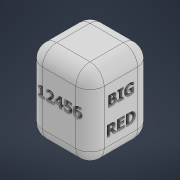
# Autodesk Inventor part: Big Red Basic Capstone
Saved by Autodesk Inventor 2022 (Build 260153000, 153)
## iProperties
Created: 2022-01-25
Part Number: Big Red Basic Capstone
Material: Generic
Document SubType Name: Modeling
Designer: izack
Density: 1 g/cm^3
Appearance: Default
Author: izack
Autodesk Inventor part; units mm, degrees
ref_plane "YZ Plane" through (0, 0, 0) normal (1, 0, 0) x (0, 1, 0)
ref_plane "XZ Plane" through (0, 0, 0) normal (0, 1, 0) x (-1, 0, 0)
ref_plane "XY Plane" through (0, 0, 0) normal (0, 0, 1) x (1, 0, 0)
sketch "Sketch1" plane through (0, 0, 0) normal (0, 1, 0) x (-1, 0, 0)
  line L0 (0, 0) -> (76.2, 0)
  line L1 (76.2, 0) -> (76.2, -76.2)
  line L2 (76.2, -76.2) -> (0, -76.2)
  line L3 (0, -76.2) -> (0, 0)
  dimension "d0" = 76.2
  dimension "d1" = 76.2
  constraints: 8 end point, 2 parallel, 1 horizontal, 1 perpendicular
  measures "d0" distance of L1.end L2.end
  measures "d1" distance of L0.end L1.end
extrude "Extrusion1" add sketch "Sketch1" along normal blind 101.6
shell "Shell1" thickness 12.7 removed faces 1 at (-25.4, 0, -25.4)
fillet "Fillet1" radius 17.4625 20 edges at (-38.1, 88.9, -63.5) (-63.5, 88.9, -38.1) (-63.5, 44.45, -63.5) (-63.5, 44.45, -12.7) (-12.7, 88.9, -38.1) (-38.1, 88.9, -12.7) (-12.7, 44.45, -63.5) (-12.7, 44.45, -12.7) (-38.1, 0, -76.2) (-76.2, 0, -38.1) (-38.1, 0, 0) (0, 0, -38.1) (-76.2, 50.8, -76.2) (-38.1, 101.6, -76.2) (-76.2, 101.6, -38.1) (0, 50.8, -76.2) (-76.2, 50.8, 0) (0, 50.8, 0) (-38.1, 101.6, 0) (0, 101.6, -38.1)
sketch "Sketch2" plane through (-76.2, 17.4625, -17.4625) normal (-1, 0, 0) x (0, 0, 1)
  line L0 (-41.275, 66.675) -> (-41.275, 0) projected
  line L1 (-41.275, 41.2843) -> (0, 41.2843)
  line L2 (0, 41.2843) -> (0, 10.1549)
  line L3 (0, 0) -> (0, 66.675) projected
  line L4 (-41.275, 10.1549) -> (0, 10.1549)
  spline S0 degree 2 poles (-25.8863, 45.1746) (-25.8863, 44.2278) (-26.6067, 42.7972) (-27.2036, 42.3238) knots 0 0 0 1 2 2 2
  spline S1 degree 2 poles (-27.2036, 42.3238) (-27.924, 41.7577) (-29.6325, 41.2843) (-30.9601, 41.2843) knots 0 0 0 1 2 2 2
  line L5 (-30.9601, 41.2843) -> (-36.0339, 41.2843)
  line L6 (-36.0339, 41.2843) -> (-36.0339, 53.9843)
  line L7 (-36.0339, 53.9843) -> (-31.557, 53.9843)
  spline S2 degree 2 poles (-31.557, 53.9843) (-30.1574, 53.9843) (-28.7165, 53.7682) (-28.0887, 53.4286) knots 0 0 0 1 2 2 2
  spline S3 degree 2 poles (-28.0887, 53.4286) (-27.3992, 53.0684) (-26.7302, 51.8333) (-26.7302, 51.0306) knots 0 0 0 1 2 2 2
  spline S4 degree 2 poles (-26.7302, 51.0306) (-26.7302, 50.1043) (-27.6565, 48.6532) (-28.4798, 48.3136) knots 0 0 0 1 2 2 2
  line L8 (-28.4798, 48.3136) -> (-28.4798, 48.2518)
  spline S5 degree 2 poles (-28.4798, 48.2518) (-27.2963, 48.0048) (-25.8863, 46.4713) (-25.8863, 45.1746) knots 0 0 0 1 2 2 2
  spline S6 degree 2 poles (-29.1796, 45.226) (-29.1796, 45.823) (-29.6531, 46.4919) (-30.1265, 46.6669) knots 0 0 0 1 2 2 2
  spline S7 degree 2 poles (-30.1265, 46.6669) (-30.4146, 46.7801) (-31.4335, 46.8007) (-32.2775, 46.8007) knots 0 0 0 1 2 2 2
  line L9 (-32.2775, 46.8007) -> (-32.8641, 46.8007)
  line L10 (-32.8641, 46.8007) -> (-32.8641, 43.6)
  line L11 (-32.8641, 43.6) -> (-32.6891, 43.6)
  spline S8 degree 2 poles (-32.6891, 43.6) (-31.4541, 43.6) (-30.5073, 43.6308) (-30.0133, 43.847) knots 0 0 0 1 2 2 2
  spline S9 degree 2 poles (-30.0133, 43.847) (-29.581, 44.0425) (-29.1796, 44.7629) (-29.1796, 45.226) knots 0 0 0 1 2 2 2
  spline S10 degree 2 poles (-29.9721, 50.4028) (-29.9721, 50.7115) (-30.2911, 51.3599) (-30.6205, 51.504) knots 0 0 0 1 2 2 2
  spline S11 degree 2 poles (-30.6205, 51.504) (-30.9292, 51.6481) (-31.7937, 51.6687) (-32.648, 51.6687) knots 0 0 0 1 2 2 2
  line L12 (-32.648, 51.6687) -> (-32.8641, 51.6687)
  line L13 (-32.8641, 51.6687) -> (-32.8641, 48.9722)
  line L14 (-32.8641, 48.9722) -> (-32.4627, 48.9722)
  spline S12 degree 2 poles (-32.4627, 48.9722) (-31.6497, 48.9722) (-30.991, 49.0031) (-30.6411, 49.1678) knots 0 0 0 1 2 2 2
  spline S13 degree 2 poles (-30.6411, 49.1678) (-30.2603, 49.353) (-29.9721, 49.9808) (-29.9721, 50.4028) knots 0 0 0 1 2 2 2
  line L15 (-17.7352, 41.2843) -> (-24.5689, 41.2843)
  line L16 (-24.5689, 41.2843) -> (-24.5689, 43.497)
  line L17 (-24.5689, 43.497) -> (-22.7473, 43.497)
  line L18 (-22.7473, 43.497) -> (-22.7473, 51.7716)
  line L19 (-22.7473, 51.7716) -> (-24.5689, 51.7716)
  line L20 (-24.5689, 51.7716) -> (-24.5689, 53.9843)
  line L21 (-24.5689, 53.9843) -> (-17.7352, 53.9843)
  line L22 (-17.7352, 53.9843) -> (-17.7352, 51.7716)
  line L23 (-17.7352, 51.7716) -> (-19.5569, 51.7716)
  line L24 (-19.5569, 51.7716) -> (-19.5569, 43.497)
  line L25 (-19.5569, 43.497) -> (-17.7352, 43.497)
  line L26 (-17.7352, 43.497) -> (-17.7352, 41.2843)
  spline S14 degree 2 poles (-5.0146, 42.0047) (-5.8483, 41.6651) (-8.5138, 41.0167) (-9.8106, 41.0167) knots 0 0 0 1 2 2 2
  spline S15 degree 2 poles (-9.8106, 41.0167) (-12.8055, 41.0167) (-16.3561, 44.4748) (-16.3561, 47.6446) knots 0 0 0 1 2 2 2
  spline S16 degree 2 poles (-16.3561, 47.6446) (-16.3561, 50.6292) (-12.8055, 54.2313) (-9.718, 54.2313) knots 0 0 0 1 2 2 2
  spline S17 degree 2 poles (-9.718, 54.2313) (-8.1228, 54.2313) (-6.1262, 53.6241) (-5.0661, 53.1095) knots 0 0 0 1 2 2 2
  line L27 (-5.0661, 53.1095) -> (-5.0661, 50.1249)
  line L28 (-5.0661, 50.1249) -> (-5.3543, 50.1249)
  spline S18 degree 2 poles (-5.3543, 50.1249) (-5.5807, 50.2999) (-6.4452, 50.9688) (-6.8569, 51.1953) knots 0 0 0 1 2 2 2
  spline S19 degree 2 poles (-6.8569, 51.1953) (-7.3303, 51.4731) (-8.5859, 51.8642) (-9.2857, 51.8642) knots 0 0 0 1 2 2 2
  spline S20 degree 2 poles (-9.2857, 51.8642) (-10.0988, 51.8642) (-11.447, 51.3496) (-11.9719, 50.8248) knots 0 0 0 1 2 2 2
  spline S21 degree 2 poles (-11.9719, 50.8248) (-12.4762, 50.3102) (-13.0628, 48.7355) (-13.0628, 47.6961) knots 0 0 0 1 2 2 2
  spline S22 degree 2 poles (-13.0628, 47.6961) (-13.0628, 45.4731) (-10.8295, 43.353) (-8.9049, 43.353) knots 0 0 0 1 2 2 2
  spline S23 degree 2 poles (-8.9049, 43.353) (-8.73, 43.353) (-8.2771, 43.3735) (-8.1022, 43.3838) knots 0 0 0 1 2 2 2
  line L29 (-8.1022, 43.3838) -> (-8.1022, 45.8847)
  line L30 (-8.1022, 45.8847) -> (-10.5619, 45.8847)
  line L31 (-10.5619, 45.8847) -> (-10.5619, 48.2621)
  line L32 (-10.5619, 48.2621) -> (-5.0146, 48.2621)
  line L33 (-5.0146, 48.2621) -> (-5.0146, 42.0047)
  line L34 (-25.912, 10.1549) -> (-29.792, 10.1549)
  line L35 (-29.792, 10.1549) -> (-33.3221, 14.817)
  line L36 (-33.3221, 14.817) -> (-34.4747, 14.817)
  line L37 (-34.4747, 14.817) -> (-34.4747, 10.1549)
  line L38 (-34.4747, 10.1549) -> (-37.6446, 10.1549)
  line L39 (-37.6446, 10.1549) -> (-37.6446, 22.8549)
  line L40 (-37.6446, 22.8549) -> (-32.5399, 22.8549)
  spline S24 degree 2 poles (-32.5399, 22.8549) (-31.4798, 22.8549) (-29.9155, 22.5873) (-29.2465, 22.1756) knots 0 0 0 1 2 2 2
  spline S25 degree 2 poles (-29.2465, 22.1756) (-28.5673, 21.7434) (-27.7645, 20.3952) (-27.7645, 19.366) knots 0 0 0 1 2 2 2
  spline S26 degree 2 poles (-27.7645, 19.366) (-27.7645, 17.9149) (-29.0819, 16.0932) (-30.1831, 15.558) knots 0 0 0 1 2 2 2
  line L41 (-30.1831, 15.558) -> (-25.912, 10.1549)
  spline S27 degree 2 poles (-31.0373, 18.9646) (-31.0373, 19.4483) (-31.4078, 20.1379) (-31.8298, 20.3231) knots 0 0 0 1 2 2 2
  spline S28 degree 2 poles (-31.8298, 20.3231) (-32.1282, 20.4466) (-32.8589, 20.5187) (-33.4044, 20.5187) knots 0 0 0 1 2 2 2
  line L42 (-33.4044, 20.5187) -> (-34.4747, 20.5187)
  line L43 (-34.4747, 20.5187) -> (-34.4747, 17.1018)
  line L44 (-34.4747, 17.1018) -> (-33.5588, 17.1018)
  spline S29 degree 2 poles (-33.5588, 17.1018) (-32.9001, 17.1018) (-31.9636, 17.2665) (-31.6445, 17.5238) knots 0 0 0 1 2 2 2
  spline S30 degree 2 poles (-31.6445, 17.5238) (-31.3358, 17.7708) (-31.0373, 18.4294) (-31.0373, 18.9646) knots 0 0 0 1 2 2 2
  line L45 (-24.9652, 10.1549) -> (-24.9652, 22.8549)
  line L46 (-24.9652, 22.8549) -> (-16.3819, 22.8549)
  line L47 (-16.3819, 22.8549) -> (-16.3819, 20.4363)
  line L48 (-16.3819, 20.4363) -> (-21.7953, 20.4363)
  line L49 (-21.7953, 20.4363) -> (-21.7953, 18.203)
  line L50 (-21.7953, 18.203) -> (-16.8038, 18.203)
  line L51 (-16.8038, 18.203) -> (-16.8038, 15.7845)
  line L52 (-16.8038, 15.7845) -> (-21.7953, 15.7845)
  line L53 (-21.7953, 15.7845) -> (-21.7953, 12.5734)
  line L54 (-21.7953, 12.5734) -> (-16.3819, 12.5734)
  line L55 (-16.3819, 12.5734) -> (-16.3819, 10.1549)
  line L56 (-16.3819, 10.1549) -> (-24.9652, 10.1549)
  spline S31 degree 2 poles (-2.8894, 16.4946) (-2.8894, 14.7141) (-4.4435, 11.9148) (-5.627, 11.1635) knots 0 0 0 1 2 2 2
  spline S32 degree 2 poles (-5.627, 11.1635) (-6.615, 10.5254) (-8.9409, 10.1549) (-10.248, 10.1549) knots 0 0 0 1 2 2 2
  line L57 (-10.248, 10.1549) -> (-14.2206, 10.1549)
  line L58 (-14.2206, 10.1549) -> (-14.2206, 22.8549)
  line L59 (-14.2206, 22.8549) -> (-10.2892, 22.8549)
  spline S33 degree 2 poles (-10.2892, 22.8549) (-8.9512, 22.8549) (-6.615, 22.5153) (-5.5858, 21.8566) knots 0 0 0 1 2 2 2
  spline S34 degree 2 poles (-5.5858, 21.8566) (-4.3405, 21.0538) (-2.8894, 18.3368) (-2.8894, 16.4946) knots 0 0 0 1 2 2 2
  spline S35 degree 2 poles (-6.1622, 16.5152) (-6.1622, 17.7708) (-7.0267, 19.5615) (-7.9118, 20.0658) knots 0 0 0 1 2 2 2
  spline S36 degree 2 poles (-7.9118, 20.0658) (-8.5602, 20.4157) (-9.9804, 20.4878) (-10.9684, 20.4878) knots 0 0 0 1 2 2 2
  line L60 (-10.9684, 20.4878) -> (-11.0302, 20.4878)
  line L61 (-11.0302, 20.4878) -> (-11.0302, 12.5323)
  line L62 (-11.0302, 12.5323) -> (-10.9684, 12.5323)
  spline S37 degree 2 poles (-10.9684, 12.5323) (-9.8981, 12.5323) (-8.4264, 12.6043) (-7.7574, 13.0263) knots 0 0 0 1 2 2 2
  spline S38 degree 2 poles (-7.7574, 13.0263) (-6.9752, 13.5203) (-6.1622, 15.2596) (-6.1622, 16.5152) knots 0 0 0 1 2 2 2
  point P0 (17.4625, -17.4625)
  constraints: 6 end point, 3 horizontal, 2 point on line, 1 perpendicular
extrude "Extrusion2" cut sketch "Sketch2" against normal blind 5.08 contours L6 L7 S2 S3 S4 L8 S5 S0 S1 L1 | L39 L40 S24 S25 S26 L41 L4 L35 L36 L37 | L16 L17 L18 L19 L20 L21 L22 L23 L24 L25 L26 L1 | S15 S16 S17 L27 L28 S18 S19 S20 S21 S22 S23 L29 L30 L31 L32 L33 S14 L1 | L1 S14 S15 | L45 L46 L47 L48 L49 L50 L51 L52 L53 L54 L55 L4 | L58 L59 S33 S34 S31 S32 L4
sketch "Sketch3" plane through (-58.7375, 17.4625, 0) normal (0, 0, 1) x (1, 0, 0)
  line L0 (0, 66.675) -> (0, 0) projected
  line L1 (0, 33.3375) -> (41.275, 33.3375)
  line L2 (41.275, 0) -> (41.275, 66.675) projected
  line L3 (2.8791, 33.3375) -> (-5.5086, 33.3375)
  line L4 (-5.5086, 33.3375) -> (-5.5086, 35.5502)
  line L5 (-5.5086, 35.5502) -> (-2.8328, 35.5502)
  line L6 (-2.8328, 35.5502) -> (-2.8328, 42.2707)
  line L7 (-2.8328, 42.2707) -> (-5.5086, 42.2707)
  line L8 (-5.5086, 42.2707) -> (-5.5086, 44.3394)
  spline S0 degree 2 poles (-5.5086, 44.3394) (-4.922, 44.3394) (-3.7591, 44.4937) (-3.4091, 44.6584) knots 0 0 0 1 2 2 2
  spline S1 degree 2 poles (-3.4091, 44.6584) (-3.0078, 44.8642) (-2.5549, 45.5538) (-2.5138, 46.0684) knots 0 0 0 1 2 2 2
  line L9 (-2.5138, 46.0684) -> (0.265, 46.0684)
  line L10 (0.265, 46.0684) -> (0.265, 35.5502)
  line L11 (0.265, 35.5502) -> (2.8791, 35.5502)
  line L12 (2.8791, 35.5502) -> (2.8791, 33.3375)
  line L13 (14.5705, 33.3375) -> (5.2359, 33.3375)
  line L14 (5.2359, 33.3375) -> (5.2359, 35.4061)
  spline S2 degree 2 poles (5.2359, 35.4061) (6.4195, 36.353) (8.3131, 38.0202) (9.0233, 38.7715) knots 0 0 0 1 2 2 2
  spline S3 degree 2 poles (9.0233, 38.7715) (9.9598, 39.7493) (10.7935, 41.2416) (10.7935, 42.0237) knots 0 0 0 1 2 2 2
  spline S4 degree 2 poles (10.7935, 42.0237) (10.7935, 42.9088) (9.7334, 43.8557) (8.7866, 43.8557) knots 0 0 0 1 2 2 2
  spline S5 degree 2 poles (8.7866, 43.8557) (8.3029, 43.8557) (7.4384, 43.6189) (6.9958, 43.4337) knots 0 0 0 1 2 2 2
  spline S6 degree 2 poles (6.9958, 43.4337) (6.5636, 43.2381) (5.946, 42.8265) (5.7917, 42.7236) knots 0 0 0 1 2 2 2
  line L15 (5.7917, 42.7236) -> (5.5447, 42.7236)
  line L16 (5.5447, 42.7236) -> (5.5447, 45.492)
  spline S7 degree 2 poles (5.5447, 45.492) (6.0798, 45.7493) (8.3646, 46.2845) (9.4247, 46.2845) knots 0 0 0 1 2 2 2
  spline S8 degree 2 poles (9.4247, 46.2845) (11.6888, 46.2845) (14.0148, 44.2673) (14.0148, 42.4457) knots 0 0 0 1 2 2 2
  spline S9 degree 2 poles (14.0148, 42.4457) (14.0148, 41.3239) (12.9547, 39.1626) (11.73, 37.9276) knots 0 0 0 1 2 2 2
  spline S10 degree 2 poles (11.73, 37.9276) (10.9581, 37.166) (9.507, 35.9825) (9.1879, 35.7355) knots 0 0 0 1 2 2 2
  line L17 (9.1879, 35.7355) -> (14.5705, 35.7355)
  line L18 (14.5705, 35.7355) -> (14.5705, 33.3375)
  line L19 (25.8503, 36.3015) -> (24.1315, 36.3015)
  line L20 (24.1315, 36.3015) -> (24.1315, 33.3066)
  line L21 (24.1315, 33.3066) -> (21.0543, 33.3066)
  line L22 (21.0543, 33.3066) -> (21.0543, 36.3015)
  line L23 (21.0543, 36.3015) -> (15.4556, 36.3015)
  line L24 (15.4556, 36.3015) -> (15.4556, 38.6686)
  line L25 (15.4556, 38.6686) -> (20.9514, 46.0375)
  line L26 (20.9514, 46.0375) -> (24.1315, 46.0375)
  line L27 (24.1315, 46.0375) -> (24.1315, 38.5863)
  line L28 (24.1315, 38.5863) -> (25.8503, 38.5863)
  line L29 (25.8503, 38.5863) -> (25.8503, 36.3015)
  line L30 (21.0543, 38.5863) -> (21.0543, 42.9088)
  line L31 (21.0543, 42.9088) -> (17.833, 38.5863)
  line L32 (17.833, 38.5863) -> (21.0543, 38.5863)
  spline S11 degree 2 poles (36.5331, 37.6394) (36.5331, 36.6411) (35.8538, 34.9533) (35.1849, 34.3461) knots 0 0 0 1 2 2 2
  spline S12 degree 2 poles (35.1849, 34.3461) (34.5159, 33.7389) (32.684, 33.0699) (31.346, 33.0699) knots 0 0 0 1 2 2 2
  spline S13 degree 2 poles (31.346, 33.0699) (29.9258, 33.0802) (27.888, 33.5433) (27.2191, 33.8418) knots 0 0 0 1 2 2 2
  line L33 (27.2191, 33.8418) -> (27.2191, 36.6103)
  line L34 (27.2191, 36.6103) -> (27.5072, 36.6103)
  spline S14 degree 2 poles (27.5072, 36.6103) (27.7542, 36.4765) (28.3512, 36.1266) (28.8349, 35.9413) knots 0 0 0 1 2 2 2
  spline S15 degree 2 poles (28.8349, 35.9413) (29.2877, 35.7663) (30.2243, 35.5296) (30.7903, 35.5296) knots 0 0 0 1 2 2 2
  spline S16 degree 2 poles (30.7903, 35.5296) (31.2843, 35.5296) (32.437, 35.7766) (32.7869, 36.106) knots 0 0 0 1 2 2 2
  spline S17 degree 2 poles (32.7869, 36.106) (33.0442, 36.3633) (33.3324, 36.9911) (33.3324, 37.5159) knots 0 0 0 1 2 2 2
  spline S18 degree 2 poles (33.3324, 37.5159) (33.3324, 37.9688) (32.9619, 38.6069) (32.6634, 38.8024) knots 0 0 0 1 2 2 2
  spline S19 degree 2 poles (32.6634, 38.8024) (32.2311, 39.0906) (30.9961, 39.2552) (30.5536, 39.2552) knots 0 0 0 1 2 2 2
  spline S20 degree 2 poles (30.5536, 39.2552) (29.8537, 39.2552) (28.5261, 39.0288) (28.0424, 38.9053) knots 0 0 0 1 2 2 2
  line L35 (28.0424, 38.9053) -> (27.7645, 38.9053)
  line L36 (27.7645, 38.9053) -> (27.7645, 46.0375)
  line L37 (27.7645, 46.0375) -> (36.1832, 46.0375)
  line L38 (36.1832, 46.0375) -> (36.1832, 43.6395)
  line L39 (36.1832, 43.6395) -> (30.78, 43.6395)
  line L40 (30.78, 43.6395) -> (30.78, 41.5297)
  spline S21 degree 2 poles (30.78, 41.5297) (31.0373, 41.5503) (31.7474, 41.5709) (31.943, 41.5709) knots 0 0 0 1 2 2 2
  spline S22 degree 2 poles (31.943, 41.5709) (32.8589, 41.5709) (34.4027, 41.2004) (35.0099, 40.8196) knots 0 0 0 1 2 2 2
  spline S23 degree 2 poles (35.0099, 40.8196) (35.7303, 40.3462) (36.5331, 38.7715) (36.5331, 37.6394) knots 0 0 0 1 2 2 2
  spline S24 degree 2 poles (47.8746, 37.66) (47.8746, 35.6531) (45.3325, 33.0699) (43.1095, 33.0699) knots 0 0 0 1 2 2 2
  spline S25 degree 2 poles (43.1095, 33.0699) (41.998, 33.0699) (40.2587, 33.708) (39.6515, 34.3358) knots 0 0 0 1 2 2 2
  spline S26 degree 2 poles (39.6515, 34.3358) (38.9311, 35.0665) (38.1592, 37.3822) (38.1592, 38.998) knots 0 0 0 1 2 2 2
  spline S27 degree 2 poles (38.1592, 38.998) (38.1592, 40.6652) (38.8796, 43.2587) (39.6926, 44.257) knots 0 0 0 1 2 2 2
  spline S28 degree 2 poles (39.6926, 44.257) (40.4645, 45.2039) (42.9757, 46.2742) (44.6944, 46.2742) knots 0 0 0 1 2 2 2
  spline S29 degree 2 poles (44.6944, 46.2742) (45.3222, 46.2742) (46.5778, 46.1095) (46.8042, 46.0581) knots 0 0 0 1 2 2 2
  line L41 (46.8042, 46.0581) -> (46.8042, 43.5675)
  line L42 (46.8042, 43.5675) -> (46.5778, 43.5675)
  spline S30 degree 2 poles (46.5778, 43.5675) (46.3514, 43.6807) (45.3222, 43.9586) (44.6636, 43.9586) knots 0 0 0 1 2 2 2
  spline S31 degree 2 poles (44.6636, 43.9586) (43.1713, 43.9586) (41.5452, 42.3839) (41.3496, 40.9225) knots 0 0 0 1 2 2 2
  spline S32 degree 2 poles (41.3496, 40.9225) (41.9774, 41.3239) (43.2639, 41.7973) (44.0769, 41.7973) knots 0 0 0 1 2 2 2
  spline S33 degree 2 poles (44.0769, 41.7973) (44.7665, 41.7973) (45.9706, 41.4268) (46.4337, 41.0769) knots 0 0 0 1 2 2 2
  spline S34 degree 2 poles (46.4337, 41.0769) (47.0924, 40.5726) (47.8746, 38.9362) (47.8746, 37.66) knots 0 0 0 1 2 2 2
  spline S35 degree 2 poles (44.1593, 35.7458) (44.4063, 36.0545) (44.6738, 36.7749) (44.6738, 37.5057) knots 0 0 0 1 2 2 2
  spline S36 degree 2 poles (44.6738, 37.5057) (44.6738, 38.1232) (44.3651, 38.9259) (44.0872, 39.1626) knots 0 0 0 1 2 2 2
  spline S37 degree 2 poles (44.0872, 39.1626) (43.799, 39.4096) (43.0889, 39.5846) (42.6875, 39.5846) knots 0 0 0 1 2 2 2
  spline S38 degree 2 poles (42.6875, 39.5846) (42.3479, 39.5846) (41.6481, 39.4096) (41.3393, 39.2861) knots 0 0 0 1 2 2 2
  spline S39 degree 2 poles (41.3393, 39.2861) (41.3393, 39.2038) (41.3187, 38.8127) (41.3187, 38.5142) knots 0 0 0 1 2 2 2
  spline S40 degree 2 poles (41.3187, 38.5142) (41.3187, 37.413) (41.6995, 36.0854) (41.998, 35.7458) knots 0 0 0 1 2 2 2
  spline S41 degree 2 poles (41.998, 35.7458) (42.2141, 35.4679) (42.7905, 35.2312) (43.0992, 35.2312) knots 0 0 0 1 2 2 2
  spline S42 degree 2 poles (43.0992, 35.2312) (43.3565, 35.2312) (43.9534, 35.4885) (44.1593, 35.7458) knots 0 0 0 1 2 2 2
  point P0 (58.7375, -17.4625)
  constraints: 2 end point, 2 midpoint, 1 horizontal
extrude "Extrusion3" cut sketch "Sketch3" against normal blind 5.08
sketch "Sketch4" plane through (0, 17.4625, -58.7375) normal (1, 0, 0) x (0, 0, -1)
  line L0 (-41.275, 41.2843) -> (0, 41.2843)
  line L1 (0, 41.2843) -> (0, 10.1549)
  line L2 (-41.275, 10.1549) -> (0, 10.1549)
  spline S0 degree 2 poles (-25.8863, 45.1746) (-25.8863, 44.2278) (-26.6067, 42.7972) (-27.2036, 42.3238) knots 0 0 0 1 2 2 2
  spline S1 degree 2 poles (-27.2036, 42.3238) (-27.924, 41.7577) (-29.6325, 41.2843) (-30.9601, 41.2843) knots 0 0 0 1 2 2 2
  line L3 (-30.9601, 41.2843) -> (-36.0339, 41.2843)
  line L4 (-36.0339, 41.2843) -> (-36.0339, 53.9843)
  line L5 (-36.0339, 53.9843) -> (-31.557, 53.9843)
  spline S2 degree 2 poles (-31.557, 53.9843) (-30.1574, 53.9843) (-28.7165, 53.7682) (-28.0887, 53.4286) knots 0 0 0 1 2 2 2
  spline S3 degree 2 poles (-28.0887, 53.4286) (-27.3992, 53.0684) (-26.7302, 51.8333) (-26.7302, 51.0306) knots 0 0 0 1 2 2 2
  spline S4 degree 2 poles (-26.7302, 51.0306) (-26.7302, 50.1043) (-27.6565, 48.6532) (-28.4798, 48.3136) knots 0 0 0 1 2 2 2
  line L6 (-28.4798, 48.3136) -> (-28.4798, 48.2518)
  spline S5 degree 2 poles (-28.4798, 48.2518) (-27.2963, 48.0048) (-25.8863, 46.4713) (-25.8863, 45.1746) knots 0 0 0 1 2 2 2
  spline S6 degree 2 poles (-29.1796, 45.226) (-29.1796, 45.823) (-29.6531, 46.4919) (-30.1265, 46.6669) knots 0 0 0 1 2 2 2
  spline S7 degree 2 poles (-30.1265, 46.6669) (-30.4146, 46.7801) (-31.4335, 46.8007) (-32.2775, 46.8007) knots 0 0 0 1 2 2 2
  line L7 (-32.2775, 46.8007) -> (-32.8641, 46.8007)
  line L8 (-32.8641, 46.8007) -> (-32.8641, 43.6)
  line L9 (-32.8641, 43.6) -> (-32.6891, 43.6)
  spline S8 degree 2 poles (-32.6891, 43.6) (-31.4541, 43.6) (-30.5073, 43.6308) (-30.0133, 43.847) knots 0 0 0 1 2 2 2
  spline S9 degree 2 poles (-30.0133, 43.847) (-29.581, 44.0425) (-29.1796, 44.7629) (-29.1796, 45.226) knots 0 0 0 1 2 2 2
  spline S10 degree 2 poles (-29.9721, 50.4028) (-29.9721, 50.7115) (-30.2911, 51.3599) (-30.6205, 51.504) knots 0 0 0 1 2 2 2
  spline S11 degree 2 poles (-30.6205, 51.504) (-30.9292, 51.6481) (-31.7937, 51.6687) (-32.648, 51.6687) knots 0 0 0 1 2 2 2
  line L10 (-32.648, 51.6687) -> (-32.8641, 51.6687)
  line L11 (-32.8641, 51.6687) -> (-32.8641, 48.9722)
  line L12 (-32.8641, 48.9722) -> (-32.4627, 48.9722)
  spline S12 degree 2 poles (-32.4627, 48.9722) (-31.6497, 48.9722) (-30.991, 49.0031) (-30.6411, 49.1678) knots 0 0 0 1 2 2 2
  spline S13 degree 2 poles (-30.6411, 49.1678) (-30.2603, 49.353) (-29.9721, 49.9808) (-29.9721, 50.4028) knots 0 0 0 1 2 2 2
  line L13 (-17.7352, 41.2843) -> (-24.5689, 41.2843)
  line L14 (-24.5689, 41.2843) -> (-24.5689, 43.497)
  line L15 (-24.5689, 43.497) -> (-22.7473, 43.497)
  line L16 (-22.7473, 43.497) -> (-22.7473, 51.7716)
  line L17 (-22.7473, 51.7716) -> (-24.5689, 51.7716)
  line L18 (-24.5689, 51.7716) -> (-24.5689, 53.9843)
  line L19 (-24.5689, 53.9843) -> (-17.7352, 53.9843)
  line L20 (-17.7352, 53.9843) -> (-17.7352, 51.7716)
  line L21 (-17.7352, 51.7716) -> (-19.5569, 51.7716)
  line L22 (-19.5569, 51.7716) -> (-19.5569, 43.497)
  line L23 (-19.5569, 43.497) -> (-17.7352, 43.497)
  line L24 (-17.7352, 43.497) -> (-17.7352, 41.2843)
  spline S14 degree 2 poles (-5.0146, 42.0047) (-5.8483, 41.6651) (-8.5138, 41.0167) (-9.8106, 41.0167) knots 0 0 0 1 2 2 2
  spline S15 degree 2 poles (-9.8106, 41.0167) (-12.8055, 41.0167) (-16.3561, 44.4748) (-16.3561, 47.6446) knots 0 0 0 1 2 2 2
  spline S16 degree 2 poles (-16.3561, 47.6446) (-16.3561, 50.6292) (-12.8055, 54.2313) (-9.718, 54.2313) knots 0 0 0 1 2 2 2
  spline S17 degree 2 poles (-9.718, 54.2313) (-8.1228, 54.2313) (-6.1262, 53.6241) (-5.0661, 53.1095) knots 0 0 0 1 2 2 2
  line L25 (-5.0661, 53.1095) -> (-5.0661, 50.1249)
  line L26 (-5.0661, 50.1249) -> (-5.3543, 50.1249)
  spline S18 degree 2 poles (-5.3543, 50.1249) (-5.5807, 50.2999) (-6.4452, 50.9688) (-6.8569, 51.1953) knots 0 0 0 1 2 2 2
  spline S19 degree 2 poles (-6.8569, 51.1953) (-7.3303, 51.4731) (-8.5859, 51.8642) (-9.2857, 51.8642) knots 0 0 0 1 2 2 2
  spline S20 degree 2 poles (-9.2857, 51.8642) (-10.0988, 51.8642) (-11.447, 51.3496) (-11.9719, 50.8248) knots 0 0 0 1 2 2 2
  spline S21 degree 2 poles (-11.9719, 50.8248) (-12.4762, 50.3102) (-13.0628, 48.7355) (-13.0628, 47.6961) knots 0 0 0 1 2 2 2
  spline S22 degree 2 poles (-13.0628, 47.6961) (-13.0628, 45.4731) (-10.8295, 43.353) (-8.9049, 43.353) knots 0 0 0 1 2 2 2
  spline S23 degree 2 poles (-8.9049, 43.353) (-8.73, 43.353) (-8.2771, 43.3735) (-8.1022, 43.3838) knots 0 0 0 1 2 2 2
  line L27 (-8.1022, 43.3838) -> (-8.1022, 45.8847)
  line L28 (-8.1022, 45.8847) -> (-10.5619, 45.8847)
  line L29 (-10.5619, 45.8847) -> (-10.5619, 48.2621)
  line L30 (-10.5619, 48.2621) -> (-5.0146, 48.2621)
  line L31 (-5.0146, 48.2621) -> (-5.0146, 42.0047)
  line L32 (-25.912, 10.1549) -> (-29.792, 10.1549)
  line L33 (-29.792, 10.1549) -> (-33.3221, 14.817)
  line L34 (-33.3221, 14.817) -> (-34.4747, 14.817)
  line L35 (-34.4747, 14.817) -> (-34.4747, 10.1549)
  line L36 (-34.4747, 10.1549) -> (-37.6446, 10.1549)
  line L37 (-37.6446, 10.1549) -> (-37.6446, 22.8549)
  line L38 (-37.6446, 22.8549) -> (-32.5399, 22.8549)
  spline S24 degree 2 poles (-32.5399, 22.8549) (-31.4798, 22.8549) (-29.9155, 22.5873) (-29.2465, 22.1756) knots 0 0 0 1 2 2 2
  spline S25 degree 2 poles (-29.2465, 22.1756) (-28.5673, 21.7434) (-27.7645, 20.3952) (-27.7645, 19.366) knots 0 0 0 1 2 2 2
  spline S26 degree 2 poles (-27.7645, 19.366) (-27.7645, 17.9149) (-29.0819, 16.0932) (-30.1831, 15.558) knots 0 0 0 1 2 2 2
  line L39 (-30.1831, 15.558) -> (-25.912, 10.1549)
  spline S27 degree 2 poles (-31.0373, 18.9646) (-31.0373, 19.4483) (-31.4078, 20.1379) (-31.8298, 20.3231) knots 0 0 0 1 2 2 2
  spline S28 degree 2 poles (-31.8298, 20.3231) (-32.1282, 20.4466) (-32.8589, 20.5187) (-33.4044, 20.5187) knots 0 0 0 1 2 2 2
  line L40 (-33.4044, 20.5187) -> (-34.4747, 20.5187)
  line L41 (-34.4747, 20.5187) -> (-34.4747, 17.1018)
  line L42 (-34.4747, 17.1018) -> (-33.5588, 17.1018)
  spline S29 degree 2 poles (-33.5588, 17.1018) (-32.9001, 17.1018) (-31.9636, 17.2665) (-31.6445, 17.5238) knots 0 0 0 1 2 2 2
  spline S30 degree 2 poles (-31.6445, 17.5238) (-31.3358, 17.7708) (-31.0373, 18.4294) (-31.0373, 18.9646) knots 0 0 0 1 2 2 2
  line L43 (-24.9652, 10.1549) -> (-24.9652, 22.8549)
  line L44 (-24.9652, 22.8549) -> (-16.3819, 22.8549)
  line L45 (-16.3819, 22.8549) -> (-16.3819, 20.4363)
  line L46 (-16.3819, 20.4363) -> (-21.7953, 20.4363)
  line L47 (-21.7953, 20.4363) -> (-21.7953, 18.203)
  line L48 (-21.7953, 18.203) -> (-16.8038, 18.203)
  line L49 (-16.8038, 18.203) -> (-16.8038, 15.7845)
  line L50 (-16.8038, 15.7845) -> (-21.7953, 15.7845)
  line L51 (-21.7953, 15.7845) -> (-21.7953, 12.5734)
  line L52 (-21.7953, 12.5734) -> (-16.3819, 12.5734)
  line L53 (-16.3819, 12.5734) -> (-16.3819, 10.1549)
  line L54 (-16.3819, 10.1549) -> (-24.9652, 10.1549)
  spline S31 degree 2 poles (-2.8894, 16.4946) (-2.8894, 14.7141) (-4.4435, 11.9148) (-5.627, 11.1635) knots 0 0 0 1 2 2 2
  spline S32 degree 2 poles (-5.627, 11.1635) (-6.615, 10.5254) (-8.9409, 10.1549) (-10.248, 10.1549) knots 0 0 0 1 2 2 2
  line L55 (-10.248, 10.1549) -> (-14.2206, 10.1549)
  line L56 (-14.2206, 10.1549) -> (-14.2206, 22.8549)
  line L57 (-14.2206, 22.8549) -> (-10.2892, 22.8549)
  spline S33 degree 2 poles (-10.2892, 22.8549) (-8.9512, 22.8549) (-6.615, 22.5153) (-5.5858, 21.8566) knots 0 0 0 1 2 2 2
  spline S34 degree 2 poles (-5.5858, 21.8566) (-4.3405, 21.0538) (-2.8894, 18.3368) (-2.8894, 16.4946) knots 0 0 0 1 2 2 2
  spline S35 degree 2 poles (-6.1622, 16.5152) (-6.1622, 17.7708) (-7.0267, 19.5615) (-7.9118, 20.0658) knots 0 0 0 1 2 2 2
  spline S36 degree 2 poles (-7.9118, 20.0658) (-8.5602, 20.4157) (-9.9804, 20.4878) (-10.9684, 20.4878) knots 0 0 0 1 2 2 2
  line L58 (-10.9684, 20.4878) -> (-11.0302, 20.4878)
  line L59 (-11.0302, 20.4878) -> (-11.0302, 12.5323)
  line L60 (-11.0302, 12.5323) -> (-10.9684, 12.5323)
  spline S37 degree 2 poles (-10.9684, 12.5323) (-9.8981, 12.5323) (-8.4264, 12.6043) (-7.7574, 13.0263) knots 0 0 0 1 2 2 2
  spline S38 degree 2 poles (-7.7574, 13.0263) (-6.9752, 13.5203) (-6.1622, 15.2596) (-6.1622, 16.5152) knots 0 0 0 1 2 2 2
  point P0 (17.4625, -17.4625)
  constraints: 6 end point, 3 horizontal, 1 perpendicular
sketch "Sketch5" plane through (-17.4625, 17.4625, -76.2) normal (0, 0, -1) x (-1, 0, 0)
  line L0 (0, 33.3375) -> (41.275, 33.3375)
  line L1 (2.8791, 33.3375) -> (-5.5086, 33.3375)
  line L2 (-5.5086, 33.3375) -> (-5.5086, 35.5502)
  line L3 (-5.5086, 35.5502) -> (-2.8328, 35.5502)
  line L4 (-2.8328, 35.5502) -> (-2.8328, 42.2707)
  line L5 (-2.8328, 42.2707) -> (-5.5086, 42.2707)
  line L6 (-5.5086, 42.2707) -> (-5.5086, 44.3394)
  spline S0 degree 2 poles (-5.5086, 44.3394) (-4.922, 44.3394) (-3.7591, 44.4937) (-3.4091, 44.6584) knots 0 0 0 1 2 2 2
  spline S1 degree 2 poles (-3.4091, 44.6584) (-3.0078, 44.8642) (-2.5549, 45.5538) (-2.5138, 46.0684) knots 0 0 0 1 2 2 2
  line L7 (-2.5138, 46.0684) -> (0.265, 46.0684)
  line L8 (0.265, 46.0684) -> (0.265, 35.5502)
  line L9 (0.265, 35.5502) -> (2.8791, 35.5502)
  line L10 (2.8791, 35.5502) -> (2.8791, 33.3375)
  line L11 (14.5705, 33.3375) -> (5.2359, 33.3375)
  line L12 (5.2359, 33.3375) -> (5.2359, 35.4061)
  spline S2 degree 2 poles (5.2359, 35.4061) (6.4195, 36.353) (8.3131, 38.0202) (9.0233, 38.7715) knots 0 0 0 1 2 2 2
  spline S3 degree 2 poles (9.0233, 38.7715) (9.9598, 39.7493) (10.7935, 41.2416) (10.7935, 42.0237) knots 0 0 0 1 2 2 2
  spline S4 degree 2 poles (10.7935, 42.0237) (10.7935, 42.9088) (9.7334, 43.8557) (8.7866, 43.8557) knots 0 0 0 1 2 2 2
  spline S5 degree 2 poles (8.7866, 43.8557) (8.3029, 43.8557) (7.4384, 43.6189) (6.9958, 43.4337) knots 0 0 0 1 2 2 2
  spline S6 degree 2 poles (6.9958, 43.4337) (6.5636, 43.2381) (5.946, 42.8265) (5.7917, 42.7236) knots 0 0 0 1 2 2 2
  line L13 (5.7917, 42.7236) -> (5.5447, 42.7236)
  line L14 (5.5447, 42.7236) -> (5.5447, 45.492)
  spline S7 degree 2 poles (5.5447, 45.492) (6.0798, 45.7493) (8.3646, 46.2845) (9.4247, 46.2845) knots 0 0 0 1 2 2 2
  spline S8 degree 2 poles (9.4247, 46.2845) (11.6888, 46.2845) (14.0148, 44.2673) (14.0148, 42.4457) knots 0 0 0 1 2 2 2
  spline S9 degree 2 poles (14.0148, 42.4457) (14.0148, 41.3239) (12.9547, 39.1626) (11.73, 37.9276) knots 0 0 0 1 2 2 2
  spline S10 degree 2 poles (11.73, 37.9276) (10.9581, 37.166) (9.507, 35.9825) (9.1879, 35.7355) knots 0 0 0 1 2 2 2
  line L15 (9.1879, 35.7355) -> (14.5705, 35.7355)
  line L16 (14.5705, 35.7355) -> (14.5705, 33.3375)
  line L17 (25.8503, 36.3015) -> (24.1315, 36.3015)
  line L18 (24.1315, 36.3015) -> (24.1315, 33.3066)
  line L19 (24.1315, 33.3066) -> (21.0543, 33.3066)
  line L20 (21.0543, 33.3066) -> (21.0543, 36.3015)
  line L21 (21.0543, 36.3015) -> (15.4556, 36.3015)
  line L22 (15.4556, 36.3015) -> (15.4556, 38.6686)
  line L23 (15.4556, 38.6686) -> (20.9514, 46.0375)
  line L24 (20.9514, 46.0375) -> (24.1315, 46.0375)
  line L25 (24.1315, 46.0375) -> (24.1315, 38.5863)
  line L26 (24.1315, 38.5863) -> (25.8503, 38.5863)
  line L27 (25.8503, 38.5863) -> (25.8503, 36.3015)
  line L28 (21.0543, 38.5863) -> (21.0543, 42.9088)
  line L29 (21.0543, 42.9088) -> (17.833, 38.5863)
  line L30 (17.833, 38.5863) -> (21.0543, 38.5863)
  spline S11 degree 2 poles (36.5331, 37.6394) (36.5331, 36.6411) (35.8538, 34.9533) (35.1849, 34.3461) knots 0 0 0 1 2 2 2
  spline S12 degree 2 poles (35.1849, 34.3461) (34.5159, 33.7389) (32.684, 33.0699) (31.346, 33.0699) knots 0 0 0 1 2 2 2
  spline S13 degree 2 poles (31.346, 33.0699) (29.9258, 33.0802) (27.888, 33.5433) (27.2191, 33.8418) knots 0 0 0 1 2 2 2
  line L31 (27.2191, 33.8418) -> (27.2191, 36.6103)
  line L32 (27.2191, 36.6103) -> (27.5072, 36.6103)
  spline S14 degree 2 poles (27.5072, 36.6103) (27.7542, 36.4765) (28.3512, 36.1266) (28.8349, 35.9413) knots 0 0 0 1 2 2 2
  spline S15 degree 2 poles (28.8349, 35.9413) (29.2877, 35.7663) (30.2243, 35.5296) (30.7903, 35.5296) knots 0 0 0 1 2 2 2
  spline S16 degree 2 poles (30.7903, 35.5296) (31.2843, 35.5296) (32.437, 35.7766) (32.7869, 36.106) knots 0 0 0 1 2 2 2
  spline S17 degree 2 poles (32.7869, 36.106) (33.0442, 36.3633) (33.3324, 36.9911) (33.3324, 37.5159) knots 0 0 0 1 2 2 2
  spline S18 degree 2 poles (33.3324, 37.5159) (33.3324, 37.9688) (32.9619, 38.6069) (32.6634, 38.8024) knots 0 0 0 1 2 2 2
  spline S19 degree 2 poles (32.6634, 38.8024) (32.2311, 39.0906) (30.9961, 39.2552) (30.5536, 39.2552) knots 0 0 0 1 2 2 2
  spline S20 degree 2 poles (30.5536, 39.2552) (29.8537, 39.2552) (28.5261, 39.0288) (28.0424, 38.9053) knots 0 0 0 1 2 2 2
  line L33 (28.0424, 38.9053) -> (27.7645, 38.9053)
  line L34 (27.7645, 38.9053) -> (27.7645, 46.0375)
  line L35 (27.7645, 46.0375) -> (36.1832, 46.0375)
  line L36 (36.1832, 46.0375) -> (36.1832, 43.6395)
  line L37 (36.1832, 43.6395) -> (30.78, 43.6395)
  line L38 (30.78, 43.6395) -> (30.78, 41.5297)
  spline S21 degree 2 poles (30.78, 41.5297) (31.0373, 41.5503) (31.7474, 41.5709) (31.943, 41.5709) knots 0 0 0 1 2 2 2
  spline S22 degree 2 poles (31.943, 41.5709) (32.8589, 41.5709) (34.4027, 41.2004) (35.0099, 40.8196) knots 0 0 0 1 2 2 2
  spline S23 degree 2 poles (35.0099, 40.8196) (35.7303, 40.3462) (36.5331, 38.7715) (36.5331, 37.6394) knots 0 0 0 1 2 2 2
  spline S24 degree 2 poles (47.8746, 37.66) (47.8746, 35.6531) (45.3325, 33.0699) (43.1095, 33.0699) knots 0 0 0 1 2 2 2
  spline S25 degree 2 poles (43.1095, 33.0699) (41.998, 33.0699) (40.2587, 33.708) (39.6515, 34.3358) knots 0 0 0 1 2 2 2
  spline S26 degree 2 poles (39.6515, 34.3358) (38.9311, 35.0665) (38.1592, 37.3822) (38.1592, 38.998) knots 0 0 0 1 2 2 2
  spline S27 degree 2 poles (38.1592, 38.998) (38.1592, 40.6652) (38.8796, 43.2587) (39.6926, 44.257) knots 0 0 0 1 2 2 2
  spline S28 degree 2 poles (39.6926, 44.257) (40.4645, 45.2039) (42.9757, 46.2742) (44.6944, 46.2742) knots 0 0 0 1 2 2 2
  spline S29 degree 2 poles (44.6944, 46.2742) (45.3222, 46.2742) (46.5778, 46.1095) (46.8042, 46.0581) knots 0 0 0 1 2 2 2
  line L39 (46.8042, 46.0581) -> (46.8042, 43.5675)
  line L40 (46.8042, 43.5675) -> (46.5778, 43.5675)
  spline S30 degree 2 poles (46.5778, 43.5675) (46.3514, 43.6807) (45.3222, 43.9586) (44.6636, 43.9586) knots 0 0 0 1 2 2 2
  spline S31 degree 2 poles (44.6636, 43.9586) (43.1713, 43.9586) (41.5452, 42.3839) (41.3496, 40.9225) knots 0 0 0 1 2 2 2
  spline S32 degree 2 poles (41.3496, 40.9225) (41.9774, 41.3239) (43.2639, 41.7973) (44.0769, 41.7973) knots 0 0 0 1 2 2 2
  spline S33 degree 2 poles (44.0769, 41.7973) (44.7665, 41.7973) (45.9706, 41.4268) (46.4337, 41.0769) knots 0 0 0 1 2 2 2
  spline S34 degree 2 poles (46.4337, 41.0769) (47.0924, 40.5726) (47.8746, 38.9362) (47.8746, 37.66) knots 0 0 0 1 2 2 2
  spline S35 degree 2 poles (44.1593, 35.7458) (44.4063, 36.0545) (44.6738, 36.7749) (44.6738, 37.5057) knots 0 0 0 1 2 2 2
  spline S36 degree 2 poles (44.6738, 37.5057) (44.6738, 38.1232) (44.3651, 38.9259) (44.0872, 39.1626) knots 0 0 0 1 2 2 2
  spline S37 degree 2 poles (44.0872, 39.1626) (43.799, 39.4096) (43.0889, 39.5846) (42.6875, 39.5846) knots 0 0 0 1 2 2 2
  spline S38 degree 2 poles (42.6875, 39.5846) (42.3479, 39.5846) (41.6481, 39.4096) (41.3393, 39.2861) knots 0 0 0 1 2 2 2
  spline S39 degree 2 poles (41.3393, 39.2861) (41.3393, 39.2038) (41.3187, 38.8127) (41.3187, 38.5142) knots 0 0 0 1 2 2 2
  spline S40 degree 2 poles (41.3187, 38.5142) (41.3187, 37.413) (41.6995, 36.0854) (41.998, 35.7458) knots 0 0 0 1 2 2 2
  spline S41 degree 2 poles (41.998, 35.7458) (42.2141, 35.4679) (42.7905, 35.2312) (43.0992, 35.2312) knots 0 0 0 1 2 2 2
  spline S42 degree 2 poles (43.0992, 35.2312) (43.3565, 35.2312) (43.9534, 35.4885) (44.1593, 35.7458) knots 0 0 0 1 2 2 2
  point P0 (58.7375, -17.4625)
  constraints: 2 end point, 1 horizontal
extrude "Extrusion4" cut sketch "Sketch4" against normal blind 5.08 contours L4 L5 S2 S3 S4 L6 S5 S0 S1 L0 | L14 L15 L16 L17 L18 L19 L20 L21 L22 L23 L24 L0 | S15 S16 S17 L25 L26 S18 S19 S20 S21 S22 S23 L27 L28 L29 L30 L31 S14 L0 | L0 S14 S15 | L37 L38 S24 S25 S26 L39 L2 L33 L34 L35 | L43 L44 L45 L46 L47 L48 L49 L50 L51 L52 L53 L2 | L56 L57 S33 S34 S31 S32 L2
extrude "Extrusion5" cut sketch "Sketch5" against normal blind 5.08
body "Solid1"
